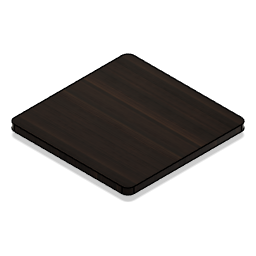
Base plate wood (Autodesk Fusion 360 design; units mm, degrees)
Autodesk Fusion 360 part; units mm, degrees
sketch "Sketch1" plane through (0, 0, 0) normal (0, 1, 0) x (1, 0, 0)
  line L0 (0, 0) -> (1000, 0)
  line L1 (1000, 0) -> (1000, -1000)
  line L2 (1000, -1000) -> (0, -1000)
  line L3 (0, -1000) -> (0, 0)
  line L4 (100, -50) -> (900, -50)
  line L5 (50, -100) -> (50, -900)
  line L6 (950, -100) -> (950, -900)
  arc A0 (100, -50) -> (50, -100) centre (100, -100) ccw
  arc A1 (950, -100) -> (900, -50) centre (900, -100) ccw
  arc A2 (50, -900) -> (100, -950) centre (100, -900) ccw
  arc A3 (903.3987, -950) -> (950, -900) centre (899.8761, -900) ccw
  line L7 (150, -100) -> (850, -100)
  line L8 (100, -150) -> (100, -850)
  line L9 (150, -900) -> (850, -900)
  line L10 (900, -150) -> (900, -850)
  arc A4 (150, -100) -> (100, -150) centre (150, -150) ccw
  arc A5 (100, -850) -> (150, -900) centre (150, -850) ccw
  arc A6 (850, -900) -> (900, -850) centre (850, -850) ccw
  arc A7 (900, -150) -> (850, -100) centre (850, -150) ccw
  line L11 (100, -950) -> (903.3987, -950)
  dimension "d2" = 1000
  dimension "d3" = 1000
  constraint coincident L0.start L3.end
  constraint horizontal L0
  constraint perpendicular L0 L1
  constraint perpendicular L1 L2
  constraint perpendicular L2 L3
  constraint perpendicular L1 L4
  constraint parallel L3 L5
  constraint perpendicular L4 L6
  constraint tangent L4 A0
  constraint tangent L4 A1
  constraint tangent L5 A2
  constraint tangent L6 A3
  constraint parallel L4 L7
  constraint perpendicular L8 L9
  constraint perpendicular L7 L10
  constraint tangent L7 A4
  constraint tangent L8 A5
  constraint tangent L10 A6
  constraint tangent L10 A7
  constraint tangent L7 A7
  constraint parallel L2 L11
  measures "d2" distance of L0.end L1.end
  measures "d3" distance of L2.end L0.start
extrude "Extrude1" add sketch "Sketch1" against normal blind 50 contours L4 L5 L6 A0 A1 A2 A3 L11
extrude "Extrude2" add sketch "Sketch1" 1 faces at (617.7996, 0, 933.3333) along normal blind 50 contours L0 L1 L2 L3 | L4 L5 L6 A0 A1 A2 A3 L11 | L7 L8 L9 L10 A4 A5 A6 A7
fillet "Fillet1" radius 50 4 edges at (0, 25, 1000) (1000, 25, 1000) (1000, 25, 0) (0, 25, 0)
